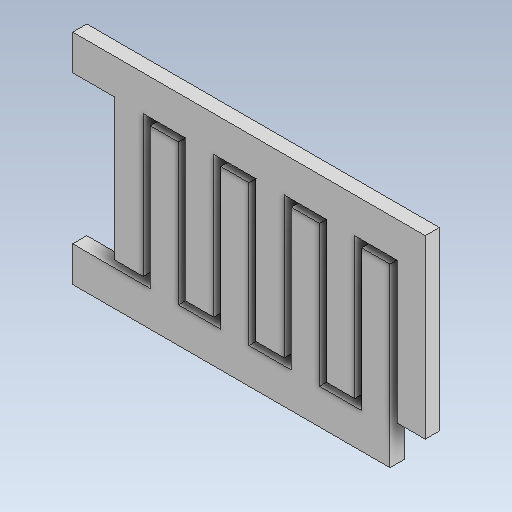
# Autodesk Inventor part: sensor-0001-002
Saved by Autodesk Inventor 2025.2 (Build 292293000, 293)
## iProperties
Created: 2025-01-19
Part Number: sensor-0001-002
Material: Genérico
Document SubType Name: Modeling
Designer: Gustavo Sousa
Density: 1 g/cm^3
Appearance: Padrão
Author: Gustavo Sousa
Autodesk Inventor part; units mm, degrees
ref_plane "YZ Plane" through (0, 0, 0) normal (1, 0, 0) x (0, 1, 0)
ref_plane "XZ Plane" through (0, 0, 0) normal (0, 1, 0) x (-1, 0, 0)
ref_plane "XY Plane" through (0, 0, 0) normal (0, 0, 1) x (1, 0, 0)
sketch "Esboço1" plane through (0, 0, 0) normal (0, 0, 1) x (1, 0, 0)
  line L0 (-25, -17.5) -> (25, -17.5) construction
  line L1 (25, 17.5) -> (-25, 17.5) construction
  line L2 (-25, -17.5) -> (25, 17.5) construction
  line L3 (25, -17.5) -> (-25, 17.5) construction
  line L4 (-25, 17.5) -> (-25, 12.5)
  line L5 (-25, 17.5) -> (25, 17.5)
  line L6 (25, 17.5) -> (25, -7.5)
  line L7 (25, -7.5) -> (21, -7.5)
  line L8 (21, -7.5) -> (21, 12.5)
  line L9 (21, 12.5) -> (15, 12.5)
  line L10 (15, 12.5) -> (15, -7.5)
  line L11 (15, -7.5) -> (11, -7.5)
  line L12 (11, -7.5) -> (11, 12.5)
  line L13 (11, 12.5) -> (5, 12.5)
  line L14 (5, 12.5) -> (5, -7.5)
  line L15 (5, -7.5) -> (1, -7.5)
  line L16 (1, -7.5) -> (1, 12.5)
  line L17 (1, 12.5) -> (-5, 12.5)
  line L18 (-5, 12.5) -> (-5, -7.5)
  line L19 (-5, -7.5) -> (-9, -7.5)
  line L20 (-9, -7.5) -> (-9, 12.5)
  line L21 (-9, 12.5) -> (-15, 12.5)
  line L22 (-15, 12.5) -> (-15, -7.5)
  line L23 (-15, -7.5) -> (-19, -7.5)
  line L24 (-19, -7.5) -> (-19, 12.5)
  line L25 (-19, 12.5) -> (-25, 12.5)
  line L26 (-25, -8.5) -> (-14, -8.5)
  line L27 (-14, -8.5) -> (-14, 11.5)
  line L28 (-14, 11.5) -> (-10, 11.5)
  line L29 (-10, 11.5) -> (-10, -8.5)
  line L30 (-10, -8.5) -> (-4, -8.5)
  line L31 (-4, -8.5) -> (-4, 11.5)
  line L32 (-4, 11.5) -> (0, 11.5)
  line L33 (0, 11.5) -> (0, -8.5)
  line L34 (0, -8.5) -> (6, -8.5)
  line L35 (6, -8.5) -> (6, 11.5)
  line L36 (6, 11.5) -> (10, 11.5)
  line L37 (10, 11.5) -> (10, -8.5)
  line L38 (10, -8.5) -> (16, -8.5)
  line L39 (16, -8.5) -> (16, 11.5)
  line L40 (16, 11.5) -> (20, 11.5)
  line L41 (25, 17.5) -> (25, -17.5) construction
  line L42 (-25, 17.5) -> (25, 17.5) construction
  line L43 (-25, -8.5) -> (-25, -13.5)
  line L44 (-25, 17.5) -> (-25, -17.5) construction
  line L45 (20, 11.5) -> (20, -13.5)
  line L46 (-25, -13.5) -> (20, -13.5)
  point P0 (0, 0)
  dimension "d2" = 35
  dimension "d3" = 5
  dimension "d17" = 6
  dimension "d18" = 4
  dimension "d23" = 50
  dimension "d25" = 25
  dimension "d27" = 5
  constraints: 94 end point, 22 horizontal alignment, 22 perpendicular, 17 point on line, 10 equal length, 9 horizontal, 9 vertical, 2 collinear, 2 midpoint, 1 parallel, 1 vertical alignment, 1 other
  measures "d2" distance of L1.end L0.start
  measures "d3" distance of L1.end L4.end
  measures "d17" distance of L8.end L9.end
  measures "d18" distance of L6.end L7.end
  measures "d23" distance of L1.start L1.end
  measures "d25" distance of L1.start L6.end
  measures "d27" distance of L26.start L43.end
extrude "Extrusão1" add sketch "Esboço1" along normal mid plane 2
